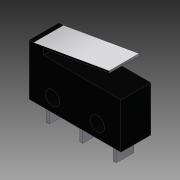
# Autodesk Inventor part: E-Stop_Zippy
Saved by Autodesk Inventor 2015 (Build 190159000, 159)
## iProperties
Created: 2015-01-06
Part Number: E-Stop_Zippy
Material: Generic
Document SubType Name: Modeling
Designer: Drew
Density: 1 g/cm^3
Appearance: Anodized - Black
Author: Drew
Autodesk Inventor part; units mm, degrees
ref_plane "YZ Plane" through (0, 0, 0) normal (1, 0, 0) x (0, 1, 0)
ref_plane "XZ Plane" through (0, 0, 0) normal (0, 1, 0) x (-1, 0, 0)
ref_plane "XY Plane" through (0, 0, 0) normal (0, 0, 1) x (1, 0, 0)
sketch "Sketch1" plane through (0, 0, 0) normal (0, 0, 1) x (1, 0, 0)
  line L0 (-9.906, -4.8895) -> (-9.906, 4.8895)
  line L1 (-6.7578, 4.8895) -> (9.906, 4.8895)
  line L2 (9.906, 4.8895) -> (9.906, -4.8895)
  line L3 (9.906, -4.8895) -> (-9.906, 4.8895) construction
  line L4 (-9.906, -4.8895) -> (9.906, 4.8895) construction
  line L5 (0, 15.8436) -> (0, -13.7401)
  line L6 (9.906, -4.8895) -> (-9.906, 4.8895) construction
  line L7 (9.906, -4.8895) -> (-9.906, -4.8895)
  line L8 (9.906, -4.8895) -> (8.255, -4.8895)
  line L9 (-9.906, 4.8895) -> (-9.906, 6.1595)
  line L10 (-9.906, 6.1595) -> (-8.9519, 6.1595)
  line L11 (-8.9519, 6.1595) -> (7.3517, 9.0343)
  line L12 (7.3517, 9.0343) -> (7.4178, 8.659)
  line L13 (7.4178, 8.659) -> (-6.7578, 6.1595)
  line L14 (-6.7578, 6.1595) -> (-6.7578, 4.8895)
  line L15 (7.4467, -4.8895) -> (0.4041, -4.8895)
  line L16 (-0.4041, -4.8895) -> (-9.906, -4.8895)
  circle A0 centre (-4.826, -2.0955) radius 1.524
  circle A1 centre (4.826, -2.0955) radius 1.524
  point P0 (0, 0)
  point P1 (-8.255, -4.8895)
  point P2 (-7.4467, -4.8895)
  point P3 (0, 0)
  point P4 (0, -9.5177)
  dimension "d4" = 9.779
  dimension "d7" = 0.381
  dimension "d8" = 10
  dimension "d9" = 19.812
  dimension "d11" = 11.049
  dimension "d16" = 3.048
  dimension "d17" = 9.652
  dimension "d18" = 2.794
  constraints: 34 end point, 8 perpendicular, 6 parallel, 6 point on line, 4 horizontal, 3 midpoint, 3 symmetric about line, 2 centre point, 1 collinear, 1 vertical, 1 other
  measures "d4" distance between parallel lines of L8 L1
  measures "d7" distance between parallel lines of L13 L11
  measures "d8" angle of L1 L13
  measures "d9" distance between parallel lines of L2 L0
  measures "d11" distance between parallel lines of L7 L10
  measures "d16" diameter of A0
  measures "d17" distance of A1.centre A0.centre
  measures "d18" distance from line of L16 A0.centre
extrude "Extrusion1" add sketch "Sketch1" along normal blind 6.4516 contours L0 L9 L10 L11 L5 L13 L14 L1 L7 | L5 L1 L2 L7 | L11 L12 L13 L5
sketch "Sketch3" plane through (-9.906, -4.8895, 0) normal (0, -1, 0) x (1, 0, 0)
  line L0 (9.906, 12.244) -> (9.906, -7.8096)
  line L1 (21.214, 3.2258) -> (-1.8957, 3.2258)
  line L2 (0, 0) -> (19.812, 0) projected
  line L3 (2.9867, 1.3208) -> (2.3517, 1.3208)
  line L4 (2.3517, 1.3208) -> (2.3517, 5.1308)
  line L5 (2.3517, 5.1308) -> (2.9867, 5.1308)
  line L6 (2.9867, 5.1308) -> (2.9867, 1.3208)
  line L7 (2.9867, 1.3208) -> (2.3517, 5.1308) construction
  line L8 (2.3517, 1.3208) -> (2.9867, 5.1308) construction
  line L9 (10.2235, 1.3208) -> (9.5885, 1.3208)
  line L10 (9.5885, 1.3208) -> (9.5885, 5.1308)
  line L11 (9.5885, 5.1308) -> (10.2235, 5.1308)
  line L12 (10.2235, 5.1308) -> (10.2235, 1.3208)
  line L13 (10.2235, 1.3208) -> (9.5885, 5.1308) construction
  line L14 (9.5885, 1.3208) -> (10.2235, 5.1308) construction
  line L15 (16.8253, 1.3208) -> (17.4603, 1.3208)
  line L16 (17.4603, 1.3208) -> (17.4603, 5.1308)
  line L17 (17.4603, 5.1308) -> (16.8253, 5.1308)
  line L18 (16.8253, 5.1308) -> (16.8253, 1.3208)
  line L19 (16.8253, 1.3208) -> (17.4603, 5.1308) construction
  line L20 (17.4603, 1.3208) -> (16.8253, 5.1308) construction
  point P0 (9.906, 0)
  point P1 (9.906, 0)
  point P2 (2.6692, 3.2258)
  point P3 (9.906, 3.2258)
  point P4 (17.1428, 3.2258)
  dimension "d19" = 0.635
  dimension "d20" = 0.635
  dimension "d21" = 3.81
  constraints: 40 end point, 7 midpoint, 5 symmetric about line, 4 parallel, 4 point on line, 3 horizontal, 2 perpendicular, 1 collinear, 1 vertical
  measures "d19" distance of L10.end L11.end
  measures "d20" distance of L4.end L5.end
  measures "d21" distance between parallel lines of L3 L5
extrude "Extrusion2" add sketch "Sketch3" along normal blind 3.81
equation "\"d20\" = d19"
body "Solid1"
